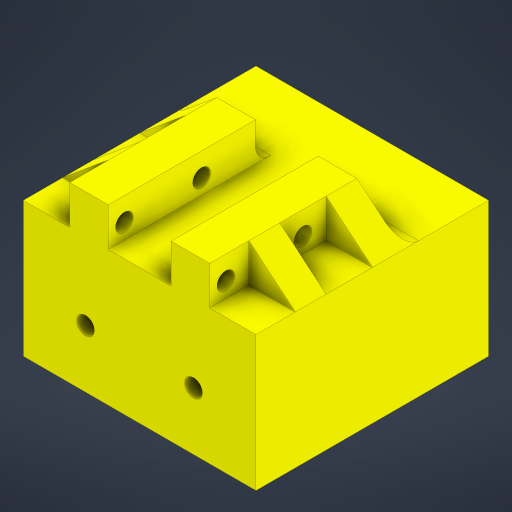
# Autodesk Inventor part: Suck-brack
Saved by Autodesk Inventor 2023 (Build 270158000, 158)
## iProperties
Created: 2023-08-09
Part Number: Suck-brack
Material: PBT Plastic
Document SubType Name: Modeling
Designer: Abhinav
Density: 1.31 g/cm^3
Appearance: Default(1)
Mass: 78.7309 g
Surface Area: 244.851 cm^2
Volume: 60.0999 cm^3
Author: Abhinav
Autodesk Inventor part; units mm, degrees
ref_plane "YZ Plane" through (0, 0, 0) normal (1, 0, 0) x (0, 1, 0)
ref_plane "XZ Plane" through (0, 0, 0) normal (0, 1, 0) x (-1, 0, 0)
sketch "Sketch1" plane through (0, 0, 0) normal (0, 1, 0) x (-1, 0, 0)
  line L0 (8.15, 22.5) -> (-8.15, 22.5)
  line L1 (-8.15, 22.5) -> (-8.15, -22.5)
  line L2 (-8.15, -22.5) -> (8.15, -22.5)
  line L3 (8.15, -22.5) -> (8.15, 22.5)
  line L4 (8.15, 22.5) -> (-8.15, -22.5) construction
  line L5 (-8.15, 22.5) -> (8.15, -22.5) construction
  line L6 (8.15, 22.5) -> (18.15, 22.5)
  line L7 (18.15, 22.5) -> (18.15, -22.5)
  line L8 (18.15, -22.5) -> (8.15, -22.5)
  line L9 (8.15, -22.5) -> (8.15, 22.5)
  line L10 (-8.15, 22.5) -> (-18.15, 22.5)
  line L11 (-18.15, 22.5) -> (-18.15, -22.5)
  line L12 (-18.15, -22.5) -> (-8.15, -22.5)
  line L13 (-8.15, -22.5) -> (-8.15, 22.5)
  line L14 (-18.15, 22.5) -> (-18.15, 15.65) construction
  line L15 (-18.15, 15.65) -> (18.15, 15.65)
  point P0 (0, 0)
  point P1 (8.15, -22.5)
  point P2 (8.15, 15.65)
  point P3 (-8.15, 15.65)
  dimension "d0" = 16.3
  dimension "d1" = 45
  dimension "d2" = 10
  dimension "d3" = 10
  dimension "d48" = 6.85
  constraints: 32 end point, 6 parallel, 4 perpendicular, 3 horizontal, 3 point on line, 2 midpoint
  measures "d0" distance of L2.end L1.end
  measures "d1" distance of L1.end L0.end
  measures "d2" distance of L7.end L8.end
  measures "d3" distance of L12.end L11.end
  measures "d48" distance of L10.end L14.end
extrude "Extrusion1" add sketch "Sketch1" along normal blind 10 contours L15 L7 L8 L3 | L1 L12 L11 L15
sketch "Sketch2" plane through (18.15, 10, 22.5) normal (1, 0, 0) x (0, 0, -1)
  line L0 (0, -10) -> (0, 0) construction
  line L1 (0, -10) -> (11, -10) construction
  line L2 (6.85, -10) -> (45, -10) construction
  line L3 (11, -10) -> (11, -6) construction
  line L4 (11, -10) -> (31, -10) construction
  line L5 (31, -10) -> (31, -6) construction
  circle A0 centre (11, -6) radius 2.25
  circle A1 centre (31, -6) radius 2.25
  point P0 (22.5, -10)
  dimension "d8" = 11
  dimension "d9" = 4
  dimension "d10" = 20
  dimension "d11" = 4
  dimension "d12" = 4.5
  constraints: 8 end point, 2 centre point, 2 coincident, 2 perpendicular, 2 point on line, 1 equal radius
  measures "d8" distance of L0.start L1.end
  measures "d9" distance of L1.end L3.end
  measures "d10" distance of L1.end L4.end
  measures "d11" distance of L4.end L5.end
  measures "d12" diameter of A0
extrude "Extrusion3" cut sketch "Sketch2" against normal blind 60
sketch "Sketch3" plane through (0, 0, 0) normal (0, -1, 0) x (1, 0, 0)
  line L0 (8.15, -22.5) -> (-8.15, -22.5) construction
  line L1 (0, -22.5) -> (0, -14.5) construction
  line L2 (-25.15, 10.65) -> (25.15, 10.65)
  line L3 (25.15, 10.65) -> (25.15, -39.65)
  line L4 (25.15, -39.65) -> (-25.15, -39.65)
  line L5 (-25.15, -39.65) -> (-25.15, 10.65)
  line L6 (-25.15, 10.65) -> (25.15, -39.65) construction
  line L7 (25.15, 10.65) -> (-25.15, -39.65) construction
  line L8 (-30.15, 15.65) -> (30.15, 15.65)
  line L9 (30.15, 15.65) -> (30.15, -44.65)
  line L10 (30.15, -44.65) -> (-30.15, -44.65)
  line L11 (-30.15, -44.65) -> (-30.15, 15.65)
  line L12 (-30.15, 15.65) -> (30.15, -44.65) construction
  line L13 (30.15, 15.65) -> (-30.15, -44.65) construction
  point P0 (0, 0)
  dimension "d16" = 8
  dimension "d17" = 50.3
  dimension "d18" = 50.3
  dimension "d19" = 60.3
  dimension "d20" = 60.3
  constraints: 26 end point, 5 midpoint, 4 parallel, 2 horizontal, 2 perpendicular, 1 vertical
  measures "d16" distance of L1.start L1.end
  measures "d17" distance of L3.end L4.end
  measures "d18" distance of L2.end L3.end
  measures "d19" distance of L9.end L10.end
  measures "d20" distance of L8.end L9.end
extrude "Extrusion4" add sketch "Sketch3" along normal blind 5 contours L2 L3 L4 L5 | L8 L9 L10 L11
extrude "Extrusion5" add sketch "Sketch3" along normal blind 35
sketch "Sketch4" plane through (30.15, 0, -44.65) normal (0, 0, -1) x (-1, 0, 0)
  circle A0 centre (44.15, -20) radius 2.25
  line L0 (16.15, -20) -> (44.15, -20) construction
  line L1 (0, -35) -> (48, -35) construction
  line L2 (0, -35) -> (0, -20) construction
  circle A1 centre (16.15, -20) radius 2.25
  line L3 (60.3, 0) -> (60.3, -35) projected
  line L4 (0, 0) -> (0, -35) projected
  line L5 (60.3, -35) -> (0, -35)
  line L6 (0, -35) -> (0, -5)
  line L7 (0, -5) -> (60.3, -5)
  line L8 (60.3, -5) -> (60.3, -35)
  line L9 (60.3, -35) -> (0, -5) construction
  line L10 (30.15, -20) -> (30.15, -16.3233) construction
  line L11 (30.15, -20) -> (30.15, -23.594) construction
  point P0 (0, -35)
  point P1 (0, -35)
  dimension "d25" = 15
  dimension "d27" = 28
  dimension "d28" = 4.5
  dimension "d29" = 4.5
  dimension "d36" = 30
  constraints: 20 end point, 2 centre point, 2 coincident, 2 midpoint, 2 parallel, 2 vertical, 1 horizontal, 1 perpendicular, 1 point on line
  measures "d25" distance of L1.start L2.end
  measures "d27" distance of L0.start L0.end
  measures "d28" diameter of A1
  measures "d29" diameter of A0
  measures "d36" distance of L5.end L6.end
extrude "Extrusion6" cut sketch "Sketch4" against normal blind 61 contours A0 | A1
sketch "Sketch5" plane through (18.15, 10, -22.5) normal (0, 0, -1) x (-1, 0, 0)
  line L0 (26.3, 0) -> (36.3, 0) projected
  line L1 (-12, -10) -> (48.3, -10) projected
  line L2 (36.3, 0) -> (36.3, -15)
  line L3 (36.3, -15) -> (48.3, -15)
  line L4 (48.3, -10) -> (36.3, 0)
  line L5 (0, -10) -> (0, 0) projected
  line L6 (0, 0) -> (0, -15)
  line L7 (-12, -10) -> (0, -10) projected
  line L8 (0, -15) -> (-12, -15)
  line L9 (-12, -10) -> (0, 0)
  point P0 (18.15, -10)
  point P1 (36.3, -10)
  constraints: 12 end point, 2 horizontal, 1 collinear, 1 vertical, 2 other
extrude "Extrusion7" add sketch "Sketch5" against normal blind 8
ref_plane "Work Plane1" through (18.15, 10, -2.5) normal (0, 0, 1) x (1, 0, 0)
sketch "Sketch6" plane through (18.15, 10, -2.5) normal (0, 0, 1) x (1, 0, 0)
  line L0 (-36.3, -10) -> (-48.3, -10) projected
  line L1 (-36.3, 0) -> (-36.3, -10) projected
  line L2 (-36.3, 0) -> (-48.3, -10) projected
  line L3 (12, -10) -> (0, -10) projected
  line L4 (12, -10) -> (0, 0) projected
  line L5 (0, -10) -> (0, 0) projected
  point P0 (-18.15, -10)
extrude "Extrusion8" add sketch "Sketch6" along normal blind 8
fillet "Fillet4" radius 4 2 edges at (19.15, 0, -22.5) (-19.15, 0, -22.5)
body "Solid1"
